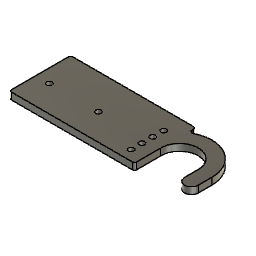
Hook v1 (Autodesk Fusion 360 design; units mm, degrees)
Autodesk Fusion 360 part; units mm, degrees
sketch "Sketch1" plane through (0, 0, 0) normal (0, 0, 1) x (1, 0, 0)
  line L0 (-13.7051, 19.3551) -> (-13.7051, 25.547)
  line L1 (-13.7051, 0.547) -> (-13.7051, -19.453)
  line L2 (-13.7051, -19.453) -> (-105.7051, -19.453)
  line L3 (-13.7051, 25.547) -> (-105.7051, 25.547)
  line L4 (-105.7051, 25.547) -> (-105.7051, -19.453)
  line L5 (13.7157, -0.0902) -> (13.7157, -10.0902)
  line L6 (23.716, -0.0313) -> (23.716, -10.0313)
  arc A0 (23.716, -0.0313) -> (-13.7051, 19.3551) centre (0, 0) ccw
  arc A1 (13.7157, -10.0313) -> (23.716, -10.0313) centre (18.7158, -10.0608) ccw
  arc A2 (13.7157, -0.0902) -> (-13.7051, -0.547) centre (0, 0) ccw
  dimension "d1" = 27.432
  dimension "d2" = 47.432
  dimension "d4" = 25
  dimension "d5" = 20
  dimension "d6" = 92
  dimension "d7" = 92
  dimension "d8" = 10
  dimension "d9" = 10
  constraint coincident A0.centre A2.centre
  constraint concentric A0 A2
  constraint coincident L1.start A2
  constraint parallel L0 L1
  constraint perpendicular L1 L2
  constraint perpendicular L0 L3
  constraint vertical L5
  constraint vertical L6
  constraint coincident L5.end A1
  constraint coincident L5 A1.start
  constraint coincident L1 A2.end
  measures "d1" diameter of A2
  measures "d2" diameter of A0
  measures "d4" distance of L1.start L0.end
  measures "d5" distance of L1.start L1.end
  measures "d6" distance of L1.end L2.end
  measures "d7" distance of L0.end L3.end
  measures "d8" distance of L5.start L5.end
  measures "d9" distance of L6.start L6.end
extrude "Extrude1" add sketch "Sketch1" along normal blind 5 contours L0 L1 L2 L3 L4 L5 L6 A0 A1 A2
fillet "Fillet1" radius 2 1 edges at (-13.7051, 19.3551, 2.5)
fillet "Fillet2" radius 1.5 1 edges at (-13.7051, 25.547, 2.5)
fillet "Fillet3" radius 1.5 1 edges at (-13.7051, -19.453, 2.5)
fillet "Fillet4" radius 1.5 2 edges at (-105.7051, 25.547, 2.5) (-105.7051, -19.453, 2.5)
sketch "Sketch2" plane through (0, 0, 5) normal (0, 0, 1) x (-1, 0, 0)
  arc A0 (105.7051, 17.953) -> (104.2051, 19.453) centre (104.2051, 17.953) ccw
  line L0 (104.2051, 19.453) -> (15.2051, 19.453)
  arc A1 (15.2051, 19.453) -> (13.7051, 17.953) centre (15.2051, 17.953) ccw
  line L1 (13.7051, 17.953) -> (13.7051, 0.547)
  arc A2 (-13.7157, 0.0902) -> (13.7051, 0.547) centre (0, 0) ccw
  line L2 (-13.7157, 0.0902) -> (-13.7157, 10.0902)
  arc A3 (-13.7157, 10.0902) -> (-23.716, 10.0313) centre (-18.7158, 10.0608) ccw
  line L3 (-23.716, 10.0313) -> (-23.716, 0.0313)
  arc A4 (-23.716, 0.0313) -> (10.7948, -21.1169) centre (0, 0) ccw
  arc A5 (13.7051, -22.8977) -> (10.7948, -21.1169) centre (11.7051, -22.8977) ccw
  line L4 (13.7051, -22.8977) -> (13.7051, -24.047)
  arc A6 (13.7051, -24.047) -> (15.2051, -25.547) centre (15.2051, -24.047) ccw
  line L5 (15.2051, -25.547) -> (104.2051, -25.547)
  arc A7 (104.2051, -25.547) -> (105.7051, -24.047) centre (104.2051, -24.047) ccw
  line L6 (105.7051, -24.047) -> (105.7051, 17.953)
  line L7 (0, 0) -> (111.4767, 0) construction
  line L8 (23.7051, -25.547) -> (23.7051, 19.453) construction
  line L9 (59.7051, -25.547) -> (59.7051, 19.453) construction
  line L10 (95.7051, -25.547) -> (95.7051, 19.453) construction
  circle A8 centre (23.7051, 12) radius 2.01
  circle A9 centre (23.7051, 4) radius 2.01
  circle A10 centre (23.7051, -12) radius 2.01
  circle A11 centre (23.7051, -4) radius 2.01
  circle A12 centre (59.7051, 0) radius 2.01
  circle A13 centre (95.7051, 0) radius 2.01
  dimension "d20" = 10
  dimension "d21" = 36
  dimension "d22" = 36
  dimension "d23" = 4.02
  dimension "d24" = 4.02
  dimension "d26" = 4.02
  dimension "d29" = 4
  dimension "d30" = 8
  dimension "d31" = 4.02
  dimension "d32" = 8
  dimension "d33" = 4
  dimension "d34" = 4.02
  dimension "d35" = 4.02
  constraint coincident A2.centre A4.centre
  constraint perpendicular L6 L7
  constraint coincident L5 L8.start
  constraint coincident L0 L8.end
  constraint perpendicular L0 L8
  constraint coincident L5 L9.start
  constraint coincident L0 L9.end
  constraint perpendicular L0 L9
  constraint coincident L5 L10.start
  constraint coincident L0 L10.end
  constraint perpendicular L0 L10
  constraint coincident L8 A8.centre
  constraint coincident L8 A9.centre
  constraint coincident L8 A10.centre
  constraint coincident L8 A11.centre
  constraint coincident L7 A12.centre
  constraint coincident L9 A12.centre
  constraint coincident L7 A13.centre
  constraint coincident L10 A13.centre
  measures "d20" distance of L1 L8
  measures "d21" distance of L8 L9
  measures "d22" distance of L9 L10
  measures "d23" diameter of A8
  measures "d24" diameter of A9
  measures "d26" diameter of A10
  measures "d29" distance of L7 A9.centre
  measures "d30" distance of A8.centre A9.centre
  measures "d31" diameter of A11
  measures "d32" distance of A10.centre A11.centre
  measures "d33" distance of L7 A11.centre
  measures "d34" diameter of A12
  measures "d35" diameter of A13
extrude "Extrude2" cut sketch "Sketch2" against normal blind 100 contours A8 | A9 | A10 | A11 | A12 | A13
